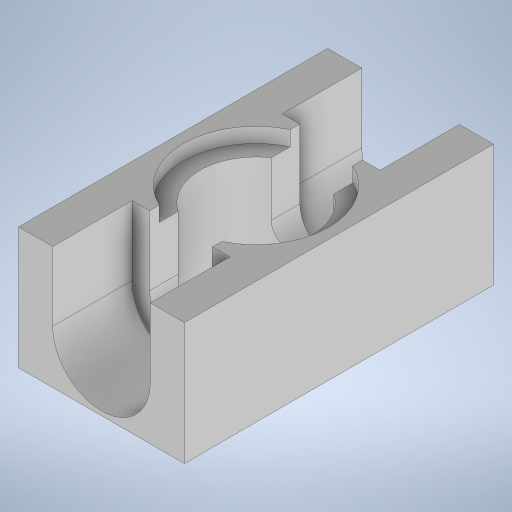
# Autodesk Inventor part: Ball Valve Mount 3
Saved by Autodesk Inventor 2024 (Build 280153000, 153)
## iProperties
Created: 2023-02-08
Part Number: Ball Valve Mount 3
Material: Generic
Document SubType Name: Modeling
Designer: tommy
Density: 1 g/cm^3
Appearance: Default
Author: tommy
Autodesk Inventor part; units mm, degrees
ref_plane "YZ Plane" through (0, 0, 0) normal (1, 0, 0) x (0, 1, 0)
ref_plane "XZ Plane" through (0, 0, 0) normal (0, 1, 0) x (-1, 0, 0)
ref_plane "XY Plane" through (0, 0, 0) normal (0, 0, 1) x (1, 0, 0)
sketch "Sketch1" plane through (0, 0, 0) normal (0, 1, 0) x (-1, 0, 0)
  circle A0 centre (0, 0) radius 8.636
  line L0 (7.5565, 23.7871) -> (-7.5565, 23.7871)
  line L1 (7.5565, -23.7871) -> (-7.5565, -23.7871)
  line L2 (7.5565, 23.7871) -> (7.5565, 8.2342)
  line L3 (7.5565, -8.2342) -> (7.5565, -23.7871)
  arc A1 (7.5565, -8.2342) -> (7.5565, 8.2342) centre (0, 0) ccw
  arc A2 (-7.5565, 8.2342) -> (-7.5565, -8.2342) centre (0, 0) ccw
  line L4 (-7.5565, -23.7871) -> (-7.5565, -8.2342)
  line L5 (-7.5565, 8.2342) -> (-7.5565, 23.7871)
  line L6 (-9.144, -8.9047) -> (-9.144, -23.7871)
  line L7 (9.144, -23.7871) -> (9.144, -8.9047)
  line L8 (7.5565, -23.7871) -> (9.144, -23.7871)
  line L9 (9.144, -23.7871) -> (-9.144, -23.7871)
  line L10 (-7.5565, 23.7871) -> (-9.144, 23.7871)
  line L11 (-9.144, 23.7871) -> (9.144, 23.7871)
  circle A3 centre (0, 0) radius 11.176
  line L12 (46.1577, 0) -> (-42.2099, 0)
  circle A4 centre (0, 0) radius 2.921 construction
  circle A5 centre (0, 0) radius 6.604 construction
  line L13 (4.7025, 16.823) -> (6.3706, 6.3706) construction
  arc A6 (4.7025, 16.823) -> (0, 20.8345) centre (0, 16.0725) ccw construction
  line L14 (-10.16, 30.48) -> (10.16, 30.48) construction
  circle A7 centre (-5.08, 34.544) radius 2.0193 construction
  line L15 (-13.97, 38.608) -> (13.97, 38.608) construction
  circle A8 centre (5.08, 34.544) radius 2.0193 construction
  line L16 (-0.508, 30.48) -> (-0.508, 38.608) construction
  line L17 (0.508, 30.48) -> (0.508, 38.608) construction
  line L18 (-10.16, -10.668) -> (-10.16, 30.48) construction
  line L19 (10.16, 9.906) -> (-10.16, 9.906) construction
  line L20 (13.97, 38.608) -> (13.97, -18.796) construction
  line L21 (-13.97, -18.796) -> (-13.97, 38.608) construction
  line L22 (10.16, 30.48) -> (10.16, -10.668) construction
  circle A9 centre (0, 0) radius 6.604 construction
  line L23 (10.16, -10.668) -> (-10.16, -10.668) construction
  circle A10 centre (5.08, -14.732) radius 2.0193 construction
  circle A11 centre (-5.08, -14.732) radius 2.0193 construction
  line L24 (-0.508, -18.796) -> (-0.508, -10.668) construction
  line L25 (0.508, -18.796) -> (0.508, -10.668) construction
  line L26 (-4.7025, -16.823) -> (-4.7191, -16.7188) construction
  line L27 (-4.7025, -16.823) -> (-4.7191, -16.7188) construction
  line L28 (13.97, -18.796) -> (-13.97, -18.796) construction
  line L29 (0, 0) -> (0, 23.3745) construction
  line L30 (-9.144, -18.796) -> (-7.5565, -18.796)
  line L31 (-9.144, -8.9047) -> (-9.144, -18.796)
  line L32 (-9.144, 23.7871) -> (-9.144, 8.9047)
  line L33 (9.144, -18.796) -> (9.144, -8.9047)
  line L34 (-12.7635, -23.7871) -> (12.7635, -23.7871)
  line L35 (12.7635, -23.7871) -> (12.7635, 23.7871)
  line L36 (12.7635, 23.7871) -> (-12.7635, 23.7871)
  line L37 (-12.7635, 23.7871) -> (-12.7635, -23.7871)
  line L38 (-12.7635, -23.7871) -> (12.7635, 23.7871) construction
  line L39 (12.7635, -23.7871) -> (-12.7635, 23.7871) construction
  circle A12 centre (0, 0) radius 12.7635
  point P0 (-7.5565, -8.2342)
  point P1 (-7.5565, 8.2342)
  point P2 (-8.636, 0)
  point P3 (8.636, 0)
  point P4 (-12.7635, 0)
  point P5 (0, 9.906)
  point P6 (-9.144, 21.9238)
  point P7 (11.176, 0)
  point P8 (-11.176, 0)
  point P9 (12.7635, 0)
  point P10 (-12.7635, 0)
  dimension "d0" = 17.272
  dimension "d6" = 15.113
  dimension "d7" = 1.5875
  dimension "d31" = 5.842
  dimension "d32" = 13.208
  dimension "d38" = 41.148
  dimension "d39" = 20.32
  dimension "d40" = 4.0386
  dimension "d41" = 4.0386
  dimension "d49" = 13.208
  constraints: 80 end point, 17 point on line, 11 centre point, 7 perpendicular, 6 parallel, 6 point on circle, 5 coincident, 5 midpoint, 3 vertical, 2 horizontal, 1 collinear, 1 concentric, 1 horizontal alignment, 5 other
  measures "d0" diameter of A0
  measures "d6" distance of L0.start L0.end
  measures "d7" distance between parallel lines of L4 L6
  measures "d31" diameter of A4
  measures "d32" diameter of A5
  measures "d38" distance of L22.start L22.end
  measures "d39" distance of L18.end L22.start
  measures "d40" diameter of A8
  measures "d41" diameter of A10
  measures "d49" diameter of A9
extrude "Extrusion1" add sketch "Sketch1" along normal blind 18.796 contours A0 L12 A2 A3 A1 | A1 L2 A12 L12 | L12 A12 L5 A2 | A3 L5 A12 L2 | A12 L2 L11 L36 L35 | L37 L36 L32 A12 | A12 L5 L0 L2 | A12 L32 L10 L5 picked at (-5.9238, 8.392)
extrude "Extrusion2" cut sketch "Sketch1" along normal blind 2.286 contours L12 A1 A3 A2 A0 | A0 L12 A2 A3 A1
sketch "Sketch2" plane through (-9.144, 0, 23.7871) normal (0, 0, 1) x (1, 0, 0)
  line L0 (9.144, 0) -> (9.144, 18.161)
  line L1 (9.144, 18.161) -> (9.144, 10.6426)
  circle A0 centre (9.144, 10.6426) radius 7.5184
  line L2 (16.6624, 10.6426) -> (16.6624, -7.5184)
  line L3 (20.32, 0) -> (-2.032, 0) projected
  line L4 (1.6256, 10.6426) -> (1.6256, -7.5184)
  line L5 (1.6256, 0) -> (16.6624, 0)
  circle A1 centre (9.144, 10.6426) radius 4.826
  line L6 (4.318, 10.6426) -> (4.318, 0)
  line L7 (13.97, 10.6426) -> (13.97, 0)
  line L8 (18.288, 0) -> (0, 0) projected
  circle A2 centre (9.144, -7.5184) radius 7.5184
  line L9 (1.6256, 10.6426) -> (16.6624, 10.6426)
  point P0 (4.318, 0)
  point P1 (4.318, 5.7651)
  point P2 (13.97, 5.7651)
  point P3 (9.144, 7.5184)
  point P4 (9.144, 0)
  dimension "d12" = 18.161
  dimension "d13" = 7.5184
  dimension "d17" = 9.652
  constraints: 16 end point, 8 point on line, 7 point on circle, 3 centre point, 3 perpendicular, 2 coincident, 2 vertical, 1 horizontal, 1 parallel
  measures "d12" distance of L0.start L0.end
  measures "d13" distance of L0.end L1.end
  measures "d17" diameter of A1
extrude "Extrusion3" cut sketch "Sketch2" against normal blind 254 contours L3 L6 A0 L0 | L0 A0 L7 L3 | A0 L6 A1 L0 | L0 A1 L7 A0 | A1 L9 L0 | L0 L9 A1 | L9 A1 L0 | L0 A1 L9
extrude "Extrusion4" cut sketch "Sketch2" against normal blind 12.2174 contours L7 A0 L2 L3 | L3 L4 A0 L6 | A0 L9 L6 | L7 L9 A0 | L9 A0 L0 A1 | A1 L0 A0 L9
mirror "Mirror3" about plane through (12.7635, 0, 0) normal (0, 0, -1)
body "Solid1"
